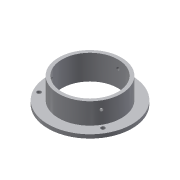
# Autodesk Inventor part: 2f1col
Saved by Autodesk Inventor 2016 (Build 200138000, 138)
## iProperties
Created: 2013-12-04
Part Number: 2f1col
Material: Aluminum 6061
Document SubType Name: Modeling
Designer: Dave
Mass: 197.234 g
Surface Area: 321.611 cm^2
Volume: 72.7802 cm^3
Density: 2.71 g/cm^3
Description: Feed mast collar
Appearance: Aluminum - Flat
Author: Dave
Autodesk Inventor part; units mm, degrees
ref_plane "YZ Plane" through (0, 0, 0) normal (1, 0, 0) x (0, 1, 0)
ref_plane "XZ Plane" through (0, 0, 0) normal (0, 1, 0) x (-1, 0, 0)
sketch "Sketch1" plane through (0, 0, 0) normal (0, 1, 0) x (-1, 0, 0)
  circle A0 centre (0, 0) radius 67.5
  dimension "d0" = 135
  constraints: 1 centre point, 1 coincident
  measures "d0" diameter of A0
extrude "body" add sketch "Sketch1" along normal blind 40
sketch "Sketch2" plane through (0, 40, 0) normal (0, 1, 0) x (1, 0, 0)
  circle A0 centre (0, 0) radius 67.5 projected
  circle A1 centre (0, 0) radius 45.085
  dimension "d4" = 90.17
  constraints: 1 centre point, 1 coincident
  measures "d4" diameter of A1
extrude "hole" cut sketch "Sketch2" against normal blind 101.6 contours A1
sketch "Sketch3" plane through (0, 40, 0) normal (0, 1, 0) x (1, 0, 0)
  circle A0 centre (0, 0) radius 45.085 projected
  circle A1 centre (0, 0) radius 67.5 projected
  circle A2 centre (0, 0) radius 50.485
  dimension "d9" = 5.4
  constraints: 1 centre point
  measures "d9" radial gap between concentric circles of A0 A2
extrude "flange" cut sketch "Sketch3" against normal blind 34 contours A1
sketch "Sketch4" plane through (0, 40, 0) normal (0, 1, 0) x (1, 0, 0)
  circle A0 centre (0, 0) radius 50.485 projected
  circle A1 centre (0, 0) radius 45.085 projected
  point P0 (0, 50.485)
  constraints: 1 vertical alignment, 1 other
ref_plane "Work Plane1" through (0, 40, -50.485) normal (0, 0, -1) x (-1, 0, 0)
sketch "Sketch5" plane through (0, 40, -50.485) normal (0, 0, -1) x (-1, 0, 0)
  circle A0 centre (0, -13) radius 2.54
  line L0 (50.485, 0) -> (-50.485, 0) projected
  point P0 (0, -40)
  dimension "d12" = 13
  dimension "d13" = 5.08
  constraints: 1 centre point
  measures "d12" distance from line of A0.centre L0
  measures "d13" diameter of A0
hole "sideHoleSE" at (0, 27, -50.485) direction (0, 0, 1) diameter 4.917 depth 17.1 tip angle 118 thread size "M6x1" class "6H" standard "ANSI Metric M Profile"
pattern_circular "sideHoleSW" count 2 over 120 about axis through (0, 40, 0) along (0, -1, 0) of "sideHoleSE"
pattern_circular "sideHoleN" count 2 over 120 about axis through (0, 40, 0) along (0, 1, 0) of "sideHoleSE"
sketch "Sketch8" plane through (0, 6, 0) normal (0, 1, 0) x (1, 0, 0)
  circle A0 centre (0, 0) radius 50.485 projected
  circle A1 centre (0, 0) radius 67.5 projected
  circle A2 centre (0, 57) radius 3.1903
  line L0 (0, 0) -> (49.3634, -28.5) construction
  line L1 (0, 0) -> (57, 0) construction
  circle A3 centre (49.3634, -28.5) radius 3.101
  line L2 (0, 0) -> (-51.9615, -30) construction
  line L3 (0, 0) -> (60, 0) construction
  circle A4 centre (-51.9615, -30) radius 3.5807
  dimension "d65" = 57
  dimension "d66" = 57
  dimension "d67" = 30
  dimension "d68" = 60
  dimension "d69" = 150
  constraints: 8 end point, 3 centre point, 2 coincident, 2 equal length, 2 horizontal
  measures "d65" distance of A0.centre A2.centre
  measures "d66" distance of L0.start L0.end
  measures "d67" angle of L0 L1
  measures "d68" distance of L0.start L2.end
  measures "d69" angle of L2 L3
hole "Hole5" at (0, 6, -57) at (49.3634, 6, 28.5) at (-51.9615, 6, 30) direction (0, -1, 0) diameter 6.6 end through all clearance for "Flat Head Machine Screw" size "M6" standard "Ansi Metric M Profile"
body "Solid1"
